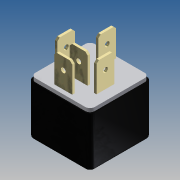
# Autodesk Inventor part: 24v relay
Saved by Autodesk Inventor 2015 SP1 (Build 190203100, 203)
## iProperties
Created: 2015-01-28
Part Number: 24v relay
Material: Acetal Resin, Black
Document SubType Name: Modeling
Designer: kevin.shaw
Mass: 21.4248 g
Surface Area: 35.5827 cm^2
Volume: 15.035 cm^3
Density: 1.425 g/cm^3
Appearance: Smooth - Black
Author: kevin.shaw
Autodesk Inventor part; units mm, degrees
note: some values were not read from the file. Chosen so that the rebuilt part matches the saved one: direction of "Emboss1".
(part 1 of 2)
ref_plane "YZ Plane" through (0, 0, 0) normal (1, 0, 0) x (0, 1, 0)
ref_plane "XZ Plane" through (0, 0, 0) normal (0, 1, 0) x (-1, 0, 0)
ref_plane "XY Plane" through (0, 0, 0) normal (0, 0, 1) x (1, 0, 0)
sketch "Sketch1" plane through (0, 0, 0) normal (0, 0, 1) x (1, 0, 0)
  line L0 (13, -13) -> (-13, -13)
  line L1 (-13, -13) -> (-13, 13)
  line L2 (-13, 13) -> (13, 13)
  line L3 (13, 13) -> (13, -13)
  line L4 (13, -13) -> (-13, 13) construction
  line L5 (-13, -13) -> (13, 13) construction
  point P0 (0, 0)
  dimension "d0" = 26
  dimension "d1" = 26
  constraints: 12 end point, 2 midpoint, 2 parallel, 1 horizontal, 1 perpendicular
  measures "d0" distance of L1.end L2.end
  measures "d1" distance of L0.end L1.end
extrude "Extrusion1" add sketch "Sketch1" along normal blind 21
sketch "Sketch2" plane through (0, 0, 21) normal (0, 0, 1) x (1, 0, 0)
  line L0 (-13, -13) -> (13, -13) projected
  line L1 (13, -13) -> (13, 13) projected
  line L2 (13, 13) -> (-13, 13) projected
  line L3 (-13, 13) -> (-13, -13) projected
  line L4 (-12.5, 12.5) -> (12.5, 12.5)
  line L5 (12.5, 12.5) -> (12.5, -12.5)
  line L6 (12.5, -12.5) -> (-12.5, -12.5)
  line L7 (-12.5, -12.5) -> (-12.5, 12.5)
  point P0 (0, 0)
  dimension "d4" = 0.5
  constraints: 8 end point, 3 other
  measures "d4" distance between parallel lines of L4 L2
extrude "Extrusion2" add sketch "Sketch2" along normal blind 1.5 contours L4 L5 L6 L7
fillet "Fillet1" radius 2 8 edges at (-13, -13, 10.5) (-13, 13, 10.5) (13, 13, 10.5) (13, -13, 10.5) (12.5, -12.5, 21.75) (-12.5, -12.5, 21.75) (-12.5, 12.5, 21.75) (12.5, 12.5, 21.75)
fillet "Fillet2" radius 1 8 edges at (12.4142, -12.4142, 0) (0, -13, 0) (-12.4142, -12.4142, 0) (-13, 0, 0) (-12.4142, 12.4142, 0) (0, 13, 0) (12.4142, 12.4142, 0) (13, 0, 0)
sketch "Sketch3" plane through (-11, 13, 21) normal (0, 1, 0) x (1, 0, 0)
  line L0 (1.1479, 5.5323) -> (24.0992, 5.5323) construction
  line L1 (24.0992, 5.5323) -> (24.0992, 1.9586) construction
  line L2 (24.0992, 1.9586) -> (1.1479, 1.9586) construction
  line L3 (1.1479, 1.9586) -> (1.1479, 5.5323) construction
  line L4 (3.2512, 2.4181) -> (1.3703, 2.4181)
  line L5 (1.3703, 2.4181) -> (1.3703, 2.8506)
  spline S0 degree 2 poles (1.3703, 2.8506) (1.573, 3.0409) (1.9338, 3.3944) (2.1069, 3.5847) knots 0 0 0 1 2 2 2
  spline S1 degree 2 poles (2.1069, 3.5847) (2.4554, 3.9678) (2.7099, 4.4275) (2.7099, 4.6722) knots 0 0 0 1 2 2 2
  spline S2 degree 2 poles (2.7099, 4.6722) (2.7099, 4.8007) (2.6308, 4.9935) (2.5592, 5.0553) knots 0 0 0 1 2 2 2
  spline S3 degree 2 poles (2.5592, 5.0553) (2.4875, 5.1171) (2.2996, 5.1789) (2.186, 5.1789) knots 0 0 0 1 2 2 2
  spline S4 degree 2 poles (2.186, 5.1789) (2.0772, 5.1789) (1.8548, 5.1245) (1.7534, 5.0825) knots 0 0 0 1 2 2 2
  spline S5 degree 2 poles (1.7534, 5.0825) (1.6669, 5.0479) (1.5063, 4.949) (1.4568, 4.9144) knots 0 0 0 1 2 2 2
  line L6 (1.4568, 4.9144) -> (1.4346, 4.9144)
  line L7 (1.4346, 4.9144) -> (1.4346, 5.3494)
  spline S6 degree 2 poles (1.4346, 5.3494) (1.5606, 5.4112) (2.0129, 5.5323) (2.2156, 5.5323) knots 0 0 0 1 2 2 2
  spline S7 degree 2 poles (2.2156, 5.5323) (2.6432, 5.5323) (3.1252, 5.08) (3.1252, 4.6945) knots 0 0 0 1 2 2 2
  spline S8 degree 2 poles (3.1252, 4.6945) (3.1252, 4.514) (3.0411, 4.2125) (2.967, 4.084) knots 0 0 0 1 2 2 2
  spline S9 degree 2 poles (2.967, 4.084) (2.8928, 3.9505) (2.6778, 3.6885) (2.5592, 3.5625) knots 0 0 0 1 2 2 2
  spline S10 degree 2 poles (2.5592, 3.5625) (2.3664, 3.3524) (1.8943, 2.9025) (1.7534, 2.7715) knots 0 0 0 1 2 2 2
  line L8 (1.7534, 2.7715) -> (3.2512, 2.7715)
  line L9 (3.2512, 2.7715) -> (3.2512, 2.4181)
  line L10 (5.6215, 3.4661) -> (5.2582, 3.4661)
  line L11 (5.2582, 3.4661) -> (5.2582, 2.4181)
  line L12 (5.2582, 2.4181) -> (4.8652, 2.4181)
  line L13 (4.8652, 2.4181) -> (4.8652, 3.4661)
  line L14 (4.8652, 3.4661) -> (3.5182, 3.4661)
  line L15 (3.5182, 3.4661) -> (3.5182, 3.8961)
  line L16 (3.5182, 3.8961) -> (4.8825, 5.4681)
  line L17 (4.8825, 5.4681) -> (5.2582, 5.4681)
  line L18 (5.2582, 5.4681) -> (5.2582, 3.7948)
  line L19 (5.2582, 3.7948) -> (5.6215, 3.7948)
  line L20 (5.6215, 3.7948) -> (5.6215, 3.4661)
  line L21 (4.8652, 3.7948) -> (4.8652, 4.9861)
  line L22 (4.8652, 4.9861) -> (3.8395, 3.7948)
  line L23 (3.8395, 3.7948) -> (4.8652, 3.7948)
  line L24 (7.8015, 4.7068) -> (6.9389, 2.4181)
  line L25 (6.9389, 2.4181) -> (6.5929, 2.4181)
  line L26 (6.5929, 2.4181) -> (5.7377, 4.7068)
  line L27 (5.7377, 4.7068) -> (6.1554, 4.7068)
  line L28 (6.1554, 4.7068) -> (6.7807, 2.9445)
  line L29 (6.7807, 2.9445) -> (7.4011, 4.7068)
  line L30 (7.4011, 4.7068) -> (7.8015, 4.7068)
  line L31 (11.7932, 2.4181) -> (11.2667, 2.4181)
  line L32 (11.2667, 2.4181) -> (10.3028, 3.6317)
  line L33 (10.3028, 3.6317) -> (9.8381, 3.6317)
  line L34 (9.8381, 3.6317) -> (9.8381, 2.4181)
  line L35 (9.8381, 2.4181) -> (9.4328, 2.4181)
  line L36 (9.4328, 2.4181) -> (9.4328, 5.4681)
  line L37 (9.4328, 5.4681) -> (10.2188, 5.4681)
  spline S11 degree 2 poles (10.2188, 5.4681) (10.4808, 5.4681) (10.8342, 5.4112) (10.9949, 5.3074) knots 0 0 0 1 2 2 2
  spline S12 degree 2 poles (10.9949, 5.3074) (11.1555, 5.2036) (11.3409, 4.8798) (11.3409, 4.6401) knots 0 0 0 1 2 2 2
  spline S13 degree 2 poles (11.3409, 4.6401) (11.3409, 4.3064) (10.9998, 3.8541) (10.7082, 3.7454) knots 0 0 0 1 2 2 2
  line L38 (10.7082, 3.7454) -> (11.7932, 2.4181)
  spline S14 degree 2 poles (10.9182, 4.608) (10.9182, 4.7414) (10.8243, 4.9466) (10.7255, 5.0133) knots 0 0 0 1 2 2 2
  spline S15 degree 2 poles (10.7255, 5.0133) (10.639, 5.0702) (10.4091, 5.1171) (10.241, 5.1171) knots 0 0 0 1 2 2 2
  line L39 (10.241, 5.1171) -> (9.8381, 5.1171)
  line L40 (9.8381, 5.1171) -> (9.8381, 3.9703)
  line L41 (9.8381, 3.9703) -> (10.1941, 3.9703)
  spline S16 degree 2 poles (10.1941, 3.9703) (10.3695, 3.9703) (10.6488, 4.0321) (10.7452, 4.1285) knots 0 0 0 1 2 2 2
  spline S17 degree 2 poles (10.7452, 4.1285) (10.8342, 4.2125) (10.9182, 4.4498) (10.9182, 4.608) knots 0 0 0 1 2 2 2
  line L42 (12.0354, 2.4181) -> (12.0354, 5.4681)
  line L43 (12.0354, 5.4681) -> (13.9435, 5.4681)
  line L44 (13.9435, 5.4681) -> (13.9435, 5.1072)
  line L45 (13.9435, 5.1072) -> (12.4408, 5.1072)
  line L46 (12.4408, 5.1072) -> (12.4408, 4.2718)
  line L47 (12.4408, 4.2718) -> (13.8422, 4.2718)
  line L48 (13.8422, 4.2718) -> (13.8422, 3.911)
  line L49 (13.8422, 3.911) -> (12.4408, 3.911)
  line L50 (12.4408, 3.911) -> (12.4408, 2.7789)
  line L51 (12.4408, 2.7789) -> (13.9435, 2.7789)
  line L52 (13.9435, 2.7789) -> (13.9435, 2.4181)
  line L53 (13.9435, 2.4181) -> (12.0354, 2.4181)
  line L54 (16.1556, 2.4181) -> (14.3884, 2.4181)
  line L55 (14.3884, 2.4181) -> (14.3884, 5.4681)
  line L56 (14.3884, 5.4681) -> (14.7938, 5.4681)
  line L57 (14.7938, 5.4681) -> (14.7938, 2.7789)
  line L58 (14.7938, 2.7789) -> (16.1556, 2.7789)
  line L59 (16.1556, 2.7789) -> (16.1556, 2.4181)
  line L60 (16.1458, 2.4181) -> (17.174, 5.4681)
  line L61 (17.174, 5.4681) -> (17.6732, 5.4681)
  line L62 (17.6732, 5.4681) -> (18.7014, 2.4181)
  line L63 (18.7014, 2.4181) -> (18.2738, 2.4181)
  line L64 (18.2738, 2.4181) -> (17.997, 3.2708)
  line L65 (17.997, 3.2708) -> (16.8329, 3.2708)
  line L66 (16.8329, 3.2708) -> (16.5561, 2.4181)
  line L67 (16.5561, 2.4181) -> (16.1458, 2.4181)
  line L68 (17.8858, 3.6168) -> (17.4137, 5.0528)
  line L69 (17.4137, 5.0528) -> (16.9441, 3.6168)
  line L70 (16.9441, 3.6168) -> (17.8858, 3.6168)
  line L71 (21.1261, 5.4681) -> (20.0954, 3.7676)
  line L72 (20.0954, 3.7676) -> (20.0954, 2.4181)
  line L73 (20.0954, 2.4181) -> (19.6901, 2.4181)
  line L74 (19.6901, 2.4181) -> (19.6901, 3.7256)
  line L75 (19.6901, 3.7256) -> (18.6594, 5.4681)
  line L76 (18.6594, 5.4681) -> (19.1093, 5.4681)
  line L77 (19.1093, 5.4681) -> (19.8952, 4.126)
  line L78 (19.8952, 4.126) -> (20.696, 5.4681)
  line L79 (20.696, 5.4681) -> (21.1261, 5.4681)
  point P0 (11, 21)
  constraints: 2 other
emboss "Emboss1" sketch "Sketch3" operation cut depth 0.1 direction (0, -1, 0)
sketch "Sketch4" plane through (0, 0, 22.5) normal (0, 0, 1) x (1, 0, 0)
  line L0 (-1.75, 11.75) -> (-0.75, 11.75)
  line L1 (-0.75, 11.75) -> (-0.75, 4.25)
  line L2 (-0.75, 4.25) -> (-1.75, 4.25)
  line L3 (-1.75, 4.25) -> (-1.75, 11.75)
  line L4 (-4.25, -3.25) -> (3.25, -3.25)
  line L5 (3.25, -3.25) -> (3.25, -4.25)
  line L6 (3.25, -4.25) -> (-4.25, -4.25)
  line L7 (-4.25, -4.25) -> (-4.25, -3.25)
  line L8 (-4.25, -9.75) -> (3.25, -9.75)
  line L9 (3.25, -9.75) -> (3.25, -10.75)
  line L10 (3.25, -10.75) -> (-4.25, -10.75)
  line L11 (-4.25, -10.75) -> (-4.25, -9.75)
  line L12 (-11, 13) -> (11, 13) projected
  line L13 (13, -11) -> (13, 11) projected
  line L14 (-9.25, 2) -> (-8.25, 2)
  line L15 (-8.25, 2) -> (-8.25, -5.5)
  line L16 (-8.25, -5.5) -> (-9.25, -5.5)
  line L17 (-9.25, -5.5) -> (-9.25, 2)
  line L18 (7.25, 2) -> (8.25, 2)
  line L19 (8.25, 2) -> (8.25, -5.5)
  line L20 (8.25, -5.5) -> (7.25, -5.5)
  line L21 (7.25, -5.5) -> (7.25, 2)
  line L22 (-13, 11) -> (-13, -11) projected
  point P0 (0, 0)
  dimension "d11" = 7.5
  dimension "d12" = 1
  dimension "d13" = 5.5
  dimension "d14" = 7.5
  dimension "d15" = 23.75
  dimension "d19" = 2.5
  dimension "d70" = 15.5
  dimension "d71" = 11.25
  dimension "d72" = 4
  dimension "d73" = 11
  constraints: 40 end point, 10 parallel, 8 equal length, 5 horizontal, 5 perpendicular, 2 point on line
  measures "d11" distance of L5.end L6.end
  measures "d12" distance of L6.end L4.start
  measures "d13" distance between parallel lines of L6 L8
  measures "d14" distance between parallel lines of L2 L4
  measures "d15" distance between parallel lines of L12 L10
  measures "d19" distance between parallel lines of L3 L7
  measures "d70" distance between parallel lines of L21 L15
  measures "d71" distance between parallel lines of L3 L22
  measures "d72" distance between parallel lines of L15 L7
  measures "d73" distance between parallel lines of L12 L18
extrude "Extrusion3" add sketch "Sketch4" along normal blind 12
chamfer "Chamfer1" distance 1 angle 45 10 edges at (-4.25, -10.25, 34.5) (3.25, -10.25, 34.5) (-4.25, -3.75, 34.5) (3.25, -3.75, 34.5) (-1.25, 4.25, 34.5) (-1.25, 11.75, 34.5) (-8.75, -5.5, 34.5) (-8.75, 2, 34.5) (7.75, -5.5, 34.5) (7.75, 2, 34.5)
hole "Hole1" at (-0.5, -10.75, 29.5) direction (0, 1, 0) diameter 2 depth 2 tip angle 118
hole "Hole2" at (-0.5, -4.25, 29.5) direction (0, 1, 0) diameter 2 depth 2 tip angle 118
hole "Hole5" at (-0.75, 8, 29.5) direction (-1, 0, 0) diameter 2 depth 2 tip angle 118
hole "Hole6" at (8.25, -1.75, 29.5) direction (-1, 0, 0) diameter 2 depth 2 tip angle 118
hole "Hole7" at (-8.25, -1.75, 29.5) direction (-1, 0, 0) diameter 2 depth 2 tip angle 118
sketch "Sketch5" plane through (0, 0, 0) normal (0, 0, -1) x (-1, 0, 0)
  line L0 (5, -5) -> (-2, -5)
  line L1 (-2, -5) -> (-2, -1)
  line L2 (-2, -1) -> (5, -1)
  line L3 (5, -1) -> (5, -5)
  line L4 (-13, 11) -> (-13, -11) projected
  line L5 (11, 13) -> (-11, 13) projected
  line L6 (3, -5) -> (0, -1)
  line L7 (8, -3) -> (6, -3)
  line L8 (7, -2.9) -> (7, 0.5)
  line L9 (7, 0.5) -> (0, 0.5)
  line L10 (7, -3) -> (6, -4.7321)
  line L11 (8, -4.7321) -> (7, -3)
  line L12 (3, -6.5) -> (7, -6.5)
  line L13 (7, -6.5) -> (7, -4.7321)
  line L14 (-2, -3) -> (-4, -3)
  line L15 (-4.9676, -7.9116) -> (-3.9257, -2.0028)
  line L16 (-3.9257, -2.0028) -> (-3.9257, 2.9972)
  line L17 (-4.8794, -7.4116) -> (-5.8794, -7.4116)
  line L18 (-5.8794, -7.4116) -> (-5.8794, -9.4116)
  line L19 (-3.3794, -7.4116) -> (-2.3794, -7.4116)
  line L20 (-2.3794, -7.4116) -> (-2.3794, -9.4116)
  line L21 (4.1535, -10.1598) -> (1.8061, -10.1598) construction
  line L22 (1.8061, -10.1598) -> (1.8061, -8.2773) construction
  line L23 (1.8061, -8.2773) -> (4.1535, -8.2773) construction
  line L24 (4.1535, -8.2773) -> (4.1535, -10.1598) construction
  line L25 (-1.2772, -11.3985) -> (-3.5284, -11.3985) construction
  line L26 (-3.5284, -11.3985) -> (-3.5284, -9.8304) construction
  line L27 (-3.5284, -9.8304) -> (-1.2772, -9.8304) construction
  line L28 (-1.2772, -9.8304) -> (-1.2772, -11.3985) construction
  line L29 (1.1157, 2.3398) -> (-1.1355, 2.3398) construction
  line L30 (-1.1355, 2.3398) -> (-1.1355, 3.9079) construction
  line L31 (-1.1355, 3.9079) -> (1.1157, 3.9079) construction
  line L32 (1.1157, 3.9079) -> (1.1157, 2.3398) construction
  line L33 (-2.7765, 3.4766) -> (-5.0277, 3.4766) construction
  line L34 (-5.0277, 3.4766) -> (-5.0277, 5.0398) construction
  line L35 (-5.0277, 5.0398) -> (-2.7765, 5.0398) construction
  line L36 (-2.7765, 5.0398) -> (-2.7765, 3.4766) construction
  line L37 (-4.4694, -11.3822) -> (-7.8036, -11.3822) construction
  line L38 (-7.8036, -11.3822) -> (-7.8036, -9.8141) construction
  line L39 (-7.8036, -9.8141) -> (-4.4694, -9.8141) construction
  line L40 (-4.4694, -9.8141) -> (-4.4694, -11.3822) construction
  line L41 (7.1, -4.7321) -> (7.1, -6.6)
  line L42 (7.1, -6.6) -> (3, -6.6)
  line L43 (8, -3) -> (8, -2.9)
  line L44 (6, -3) -> (6, -2.9)
  line L45 (7.1, -2.9) -> (7.1, 0.6)
  line L46 (7.1, 0.6) -> (0, 0.6)
  line L47 (8, -2.9) -> (7.1, -2.9)
  line L48 (7, -2.9) -> (6, -2.9)
  line L49 (-0.125, -1) -> (2.875, -5)
  line L50 (0, 2) -> (-0.1, 2)
  line L51 (3, -8) -> (2.9, -8)
  line L52 (5.1, -0.9) -> (-2.1, -0.9)
  line L53 (-2.1, -0.9) -> (-2.1, -5.1)
  line L54 (-2.1, -5.1) -> (5.1, -5.1)
  line L55 (5.1, -5.1) -> (5.1, -0.9)
  line L56 (-2.4794, -9.4116) -> (-2.4794, -7.5116)
  line L57 (-2.4794, -7.5116) -> (-3.3794, -7.5116)
  line L58 (-2.3794, -9.4116) -> (-2.4794, -9.4116)
  line L59 (-3.3794, -7.5116) -> (-3.3794, -7.4116)
  line L60 (-5.9794, -9.4116) -> (-5.9794, -7.3116)
  line L61 (-5.9794, -7.3116) -> (-4.8618, -7.3116)
  line L62 (-5.8794, -9.4116) -> (-5.9794, -9.4116)
  line L63 (-4.8691, -7.929) -> (-3.8257, -2.0115)
  line L64 (-3.8257, -2.0115) -> (-3.8257, 2.9972)
  line L65 (-4.8691, -7.929) -> (-4.9676, -7.9116)
  line L66 (-3.8257, 2.9972) -> (-3.9257, 2.9972)
  line L67 (0, 0.6) -> (0, 2)
  line L68 (3, -6.6) -> (3, -8)
  line L69 (6, -4.7321) -> (7, -4.7321)
  line L70 (7.1, -4.7321) -> (8, -4.7321)
  line L71 (3, -5.2) -> (2.9, -5.2)
  line L72 (2.9, -5.2) -> (2.9, -8)
  line L73 (3, -5.2) -> (3, -6.5)
  line L74 (0, -0.8) -> (-0.1, -0.8)
  line L75 (-0.1, 2) -> (-0.1, -0.8)
  line L76 (0, -1) -> (0, -0.9)
  line L77 (0, -0.8) -> (0, 0.5)
  line L78 (-2, -3.1) -> (-4.0176, -3.1)
  spline S0 degree 2 poles (-5.0322, -9.8141) (-4.9203, -9.8141) (-4.7368, -9.881) (-4.6724, -9.943) knots 0 0 0 1 2 2 2
  spline S1 degree 2 poles (-4.6724, -9.943) (-4.6091, -10.0038) (-4.5435, -10.1691) (-4.5435, -10.2627) knots 0 0 0 1 2 2 2
  spline S2 degree 2 poles (-4.5435, -10.2627) (-4.5435, -10.3842) (-4.6736, -10.5884) (-4.7976, -10.6492) knots 0 0 0 1 2 2 2
  line L79 (-4.7976, -10.6492) -> (-4.7976, -10.6553)
  spline S3 degree 2 poles (-4.7976, -10.6553) (-4.6869, -10.7197) (-4.58, -10.8729) (-4.58, -10.9872) knots 0 0 0 1 2 2 2
  spline S4 degree 2 poles (-4.58, -10.9872) (-4.58, -11.1561) (-4.8352, -11.3822) (-5.0322, -11.3822) knots 0 0 0 1 2 2 2
  spline S5 degree 2 poles (-5.0322, -11.3822) (-5.2364, -11.3822) (-5.4831, -11.1683) (-5.4831, -11.0005) knots 0 0 0 1 2 2 2
  spline S6 degree 2 poles (-5.4831, -11.0005) (-5.4831, -10.8996) (-5.3652, -10.7027) (-5.2546, -10.6468) knots 0 0 0 1 2 2 2
  line L80 (-5.2546, -10.6468) -> (-5.2546, -10.6407)
  spline S7 degree 2 poles (-5.2546, -10.6407) (-5.3859, -10.5799) (-5.5208, -10.4049) (-5.5208, -10.2663) knots 0 0 0 1 2 2 2
  spline S8 degree 2 poles (-5.5208, -10.2663) (-5.5208, -10.0743) (-5.2412, -9.8141) (-5.0322, -9.8141) knots 0 0 0 1 2 2 2
  spline S9 degree 2 poles (-5.3142, -10.2469) (-5.3142, -10.3393) (-5.2412, -10.4487) (-5.1379, -10.5046) knots 0 0 0 1 2 2 2
  spline S10 degree 2 poles (-5.1379, -10.5046) (-5.1039, -10.524) (-4.9896, -10.569) (-4.9179, -10.5982) knots 0 0 0 1 2 2 2
  spline S11 degree 2 poles (-4.9179, -10.5982) (-4.8352, -10.5435) (-4.7465, -10.3806) (-4.7465, -10.2773) knots 0 0 0 1 2 2 2
  spline S12 degree 2 poles (-4.7465, -10.2773) (-4.7465, -10.1411) (-4.9106, -9.9637) (-5.0346, -9.9637) knots 0 0 0 1 2 2 2
  spline S13 degree 2 poles (-5.0346, -9.9637) (-5.161, -9.9637) (-5.3142, -10.1156) (-5.3142, -10.2469) knots 0 0 0 1 2 2 2
  spline S14 degree 2 poles (-5.2862, -10.9981) (-5.2862, -11.099) (-5.1513, -11.2339) (-5.0309, -11.2339) knots 0 0 0 1 2 2 2
  spline S15 degree 2 poles (-5.0309, -11.2339) (-4.9215, -11.2339) (-4.7818, -11.1136) (-4.7818, -11.0102) knots 0 0 0 1 2 2 2
  spline S16 degree 2 poles (-4.7818, -11.0102) (-4.7818, -10.9361) (-4.8535, -10.8328) (-4.9252, -10.7914) knots 0 0 0 1 2 2 2
  spline S17 degree 2 poles (-4.9252, -10.7914) (-4.9556, -10.7744) (-5.0844, -10.7149) (-5.1367, -10.6978) knots 0 0 0 1 2 2 2
  spline S18 degree 2 poles (-5.1367, -10.6978) (-5.2242, -10.7647) (-5.2862, -10.9069) (-5.2862, -10.9981) knots 0 0 0 1 2 2 2
  line L81 (-6.6464, -11.1233) -> (-5.9973, -9.8482)
  line L82 (-5.9973, -9.8482) -> (-5.7834, -9.8482)
  line L83 (-5.7834, -9.8482) -> (-6.4689, -11.1719)
  line L84 (-6.4689, -11.1719) -> (-5.6946, -11.1719)
  line L85 (-5.6946, -11.1719) -> (-5.6946, -11.3482)
  line L86 (-5.6946, -11.3482) -> (-6.6464, -11.3482)
  line L87 (-6.6464, -11.3482) -> (-6.6464, -11.1233)
  spline S19 degree 2 poles (-7.4852, -9.9673) (-7.4621, -9.9503) (-7.3843, -9.8895) (-7.3478, -9.8713) knots 0 0 0 1 2 2 2
  spline S20 degree 2 poles (-7.3478, -9.8713) (-7.298, -9.8445) (-7.2044, -9.8166) (-7.1193, -9.8166) knots 0 0 0 1 2 2 2
  spline S21 degree 2 poles (-7.1193, -9.8166) (-7.05, -9.8166) (-6.9248, -9.8688) (-6.8774, -9.9162) knots 0 0 0 1 2 2 2
  spline S22 degree 2 poles (-6.8774, -9.9162) (-6.8324, -9.9624) (-6.7777, -10.0986) (-6.7777, -10.1739) knots 0 0 0 1 2 2 2
  spline S23 degree 2 poles (-6.7777, -10.1739) (-6.7777, -10.2906) (-6.8762, -10.456) (-6.9831, -10.5034) knots 0 0 0 1 2 2 2
  spline S24 degree 2 poles (-6.9831, -10.5034) (-7.0779, -10.5471) (-7.3356, -10.5799) (-7.4852, -10.5884) knots 0 0 0 1 2 2 2
  line L88 (-7.4852, -10.5884) -> (-7.4852, -10.6249)
  spline S25 degree 2 poles (-7.4852, -10.6249) (-7.4852, -10.6906) (-7.445, -10.772) (-7.4086, -10.7951) knots 0 0 0 1 2 2 2
  spline S26 degree 2 poles (-7.4086, -10.7951) (-7.3721, -10.8182) (-7.2676, -10.8328) (-7.2117, -10.8328) knots 0 0 0 1 2 2 2
  spline S27 degree 2 poles (-7.2117, -10.8328) (-7.146, -10.8328) (-6.9685, -10.7939) (-6.8798, -10.7562) knots 0 0 0 1 2 2 2
  line L89 (-6.8798, -10.7562) -> (-6.8689, -10.7562)
  line L90 (-6.8689, -10.7562) -> (-6.8689, -10.9495)
  spline S28 degree 2 poles (-6.8689, -10.9495) (-6.9211, -10.9641) (-7.1168, -11.0005) (-7.2129, -11.0005) knots 0 0 0 1 2 2 2
  spline S29 degree 2 poles (-7.2129, -11.0005) (-7.3296, -11.0005) (-7.4888, -10.9641) (-7.552, -10.9166) knots 0 0 0 1 2 2 2
  spline S30 degree 2 poles (-7.552, -10.9166) (-7.614, -10.8705) (-7.6748, -10.7234) (-7.6748, -10.6176) knots 0 0 0 1 2 2 2
  line L91 (-7.6748, -10.6176) -> (-7.6748, -9.8482)
  line L92 (-7.6748, -9.8482) -> (-7.4852, -9.8482)
  line L93 (-7.4852, -9.8482) -> (-7.4852, -9.9673)
  line L94 (-7.4852, -10.1253) -> (-7.4852, -10.4377)
  spline S31 degree 2 poles (-7.4852, -10.4377) (-7.4171, -10.4316) (-7.2117, -10.411) (-7.1472, -10.3915) knots 0 0 0 1 2 2 2
  spline S32 degree 2 poles (-7.1472, -10.3915) (-7.0719, -10.3684) (-6.9734, -10.2724) (-6.9734, -10.1873) knots 0 0 0 1 2 2 2
  spline S33 degree 2 poles (-6.9734, -10.1873) (-6.9734, -10.0901) (-7.0828, -9.9916) (-7.1873, -9.9916) knots 0 0 0 1 2 2 2
  spline S34 degree 2 poles (-7.1873, -9.9916) (-7.2761, -9.9916) (-7.4219, -10.0682) (-7.4852, -10.1253) knots 0 0 0 1 2 2 2
  spline S35 degree 2 poles (-1.84, -9.8304) (-1.7282, -9.8304) (-1.5446, -9.8973) (-1.4802, -9.9593) knots 0 0 0 1 2 2 2
  spline S36 degree 2 poles (-1.4802, -9.9593) (-1.417, -10.02) (-1.3513, -10.1854) (-1.3513, -10.279) knots 0 0 0 1 2 2 2
  spline S37 degree 2 poles (-1.3513, -10.279) (-1.3513, -10.4005) (-1.4814, -10.6047) (-1.6054, -10.6655) knots 0 0 0 1 2 2 2
  line L95 (-1.6054, -10.6655) -> (-1.6054, -10.6716)
  spline S38 degree 2 poles (-1.6054, -10.6716) (-1.4948, -10.736) (-1.3878, -10.8892) (-1.3878, -11.0034) knots 0 0 0 1 2 2 2
  spline S39 degree 2 poles (-1.3878, -11.0034) (-1.3878, -11.1724) (-1.6431, -11.3985) (-1.84, -11.3985) knots 0 0 0 1 2 2 2
  spline S40 degree 2 poles (-1.84, -11.3985) (-2.0442, -11.3985) (-2.291, -11.1845) (-2.291, -11.0168) knots 0 0 0 1 2 2 2
  spline S41 degree 2 poles (-2.291, -11.0168) (-2.291, -10.9159) (-2.1731, -10.719) (-2.0624, -10.6631) knots 0 0 0 1 2 2 2
  line L96 (-2.0624, -10.6631) -> (-2.0624, -10.657)
  spline S42 degree 2 poles (-2.0624, -10.657) (-2.1937, -10.5962) (-2.3286, -10.4212) (-2.3286, -10.2826) knots 0 0 0 1 2 2 2
  spline S43 degree 2 poles (-2.3286, -10.2826) (-2.3286, -10.0905) (-2.0491, -9.8304) (-1.84, -9.8304) knots 0 0 0 1 2 2 2
  spline S44 degree 2 poles (-2.122, -10.2631) (-2.122, -10.3555) (-2.0491, -10.4649) (-1.9457, -10.5208) knots 0 0 0 1 2 2 2
  spline S45 degree 2 poles (-1.9457, -10.5208) (-1.9117, -10.5403) (-1.7974, -10.5853) (-1.7257, -10.6144) knots 0 0 0 1 2 2 2
  spline S46 degree 2 poles (-1.7257, -10.6144) (-1.6431, -10.5597) (-1.5543, -10.3969) (-1.5543, -10.2935) knots 0 0 0 1 2 2 2
  spline S47 degree 2 poles (-1.5543, -10.2935) (-1.5543, -10.1574) (-1.7184, -9.9799) (-1.8424, -9.9799) knots 0 0 0 1 2 2 2
  spline S48 degree 2 poles (-1.8424, -9.9799) (-1.9688, -9.9799) (-2.122, -10.1319) (-2.122, -10.2631) knots 0 0 0 1 2 2 2
  spline S49 degree 2 poles (-2.094, -11.0144) (-2.094, -11.1153) (-1.9591, -11.2502) (-1.8388, -11.2502) knots 0 0 0 1 2 2 2
  spline S50 degree 2 poles (-1.8388, -11.2502) (-1.7294, -11.2502) (-1.5896, -11.1298) (-1.5896, -11.0265) knots 0 0 0 1 2 2 2
  spline S51 degree 2 poles (-1.5896, -11.0265) (-1.5896, -10.9524) (-1.6613, -10.849) (-1.733, -10.8077) knots 0 0 0 1 2 2 2
  spline S52 degree 2 poles (-1.733, -10.8077) (-1.7634, -10.7907) (-1.8923, -10.7311) (-1.9445, -10.7141) knots 0 0 0 1 2 2 2
  spline S53 degree 2 poles (-1.9445, -10.7141) (-2.032, -10.781) (-2.094, -10.9232) (-2.094, -11.0144) knots 0 0 0 1 2 2 2
  line L97 (-3.4543, -11.1396) -> (-2.8051, -9.8644)
  line L98 (-2.8051, -9.8644) -> (-2.5912, -9.8644)
  line L99 (-2.5912, -9.8644) -> (-3.2768, -11.1882)
  line L100 (-3.2768, -11.1882) -> (-2.5025, -11.1882)
  line L101 (-2.5025, -11.1882) -> (-2.5025, -11.3644)
  line L102 (-2.5025, -11.3644) -> (-3.4543, -11.3644)
  line L103 (-3.4543, -11.3644) -> (-3.4543, -11.1396)
  spline S54 degree 2 poles (3.5907, -8.5918) (3.7025, -8.5918) (3.8861, -8.6586) (3.9505, -8.7206) knots 0 0 0 1 2 2 2
  spline S55 degree 2 poles (3.9505, -8.7206) (4.0137, -8.7814) (4.0793, -8.9467) (4.0793, -9.0403) knots 0 0 0 1 2 2 2
  spline S56 degree 2 poles (4.0793, -9.0403) (4.0793, -9.1619) (3.9493, -9.3661) (3.8253, -9.4269) knots 0 0 0 1 2 2 2
  line L104 (3.8253, -9.4269) -> (3.8253, -9.4329)
  spline S57 degree 2 poles (3.8253, -9.4329) (3.9359, -9.4974) (4.0429, -9.6505) (4.0429, -9.7648) knots 0 0 0 1 2 2 2
  spline S58 degree 2 poles (4.0429, -9.7648) (4.0429, -9.9338) (3.7876, -10.1598) (3.5907, -10.1598) knots 0 0 0 1 2 2 2
  spline S59 degree 2 poles (3.5907, -10.1598) (3.3865, -10.1598) (3.1397, -9.9459) (3.1397, -9.7782) knots 0 0 0 1 2 2 2
  spline S60 degree 2 poles (3.1397, -9.7782) (3.1397, -9.6773) (3.2576, -9.4803) (3.3682, -9.4244) knots 0 0 0 1 2 2 2
  line L105 (3.3682, -9.4244) -> (3.3682, -9.4184)
  spline S61 degree 2 poles (3.3682, -9.4184) (3.2369, -9.3576) (3.102, -9.1825) (3.102, -9.044) knots 0 0 0 1 2 2 2
  spline S62 degree 2 poles (3.102, -9.044) (3.102, -8.8519) (3.3816, -8.5918) (3.5907, -8.5918) knots 0 0 0 1 2 2 2
  spline S63 degree 2 poles (3.3087, -9.0245) (3.3087, -9.1169) (3.3816, -9.2263) (3.4849, -9.2822) knots 0 0 0 1 2 2 2
  spline S64 degree 2 poles (3.4849, -9.2822) (3.519, -9.3017) (3.6332, -9.3466) (3.7049, -9.3758) knots 0 0 0 1 2 2 2
  spline S65 degree 2 poles (3.7049, -9.3758) (3.7876, -9.3211) (3.8763, -9.1582) (3.8763, -9.0549) knots 0 0 0 1 2 2 2
  spline S66 degree 2 poles (3.8763, -9.0549) (3.8763, -8.9188) (3.7122, -8.7413) (3.5882, -8.7413) knots 0 0 0 1 2 2 2
  spline S67 degree 2 poles (3.5882, -8.7413) (3.4618, -8.7413) (3.3087, -8.8932) (3.3087, -9.0245) knots 0 0 0 1 2 2 2
  spline S68 degree 2 poles (3.3366, -9.7757) (3.3366, -9.8766) (3.4715, -10.0115) (3.5919, -10.0115) knots 0 0 0 1 2 2 2
  spline S69 degree 2 poles (3.5919, -10.0115) (3.7013, -10.0115) (3.8411, -9.8912) (3.8411, -9.7879) knots 0 0 0 1 2 2 2
  spline S70 degree 2 poles (3.8411, -9.7879) (3.8411, -9.7137) (3.7694, -9.6104) (3.6976, -9.5691) knots 0 0 0 1 2 2 2
  spline S71 degree 2 poles (3.6976, -9.5691) (3.6672, -9.5521) (3.5384, -9.4925) (3.4861, -9.4755) knots 0 0 0 1 2 2 2
  spline S72 degree 2 poles (3.4861, -9.4755) (3.3986, -9.5423) (3.3366, -9.6846) (3.3366, -9.7757) knots 0 0 0 1 2 2 2
  spline S73 degree 2 poles (2.0092, -9.1023) (2.0092, -8.9941) (2.0785, -8.8094) (2.1417, -8.7413) knots 0 0 0 1 2 2 2
  spline S74 degree 2 poles (2.1417, -8.7413) (2.2049, -8.6732) (2.3933, -8.5942) (2.51, -8.5942) knots 0 0 0 1 2 2 2
  spline S75 degree 2 poles (2.51, -8.5942) (2.617, -8.5942) (2.8261, -8.6416) (2.9027, -8.6793) knots 0 0 0 1 2 2 2
  line L106 (2.9027, -8.6793) -> (2.9027, -8.892)
  line L107 (2.9027, -8.892) -> (2.8881, -8.892)
  spline S76 degree 2 poles (2.8881, -8.892) (2.865, -8.875) (2.7787, -8.8312) (2.7264, -8.8118) knots 0 0 0 1 2 2 2
  spline S77 degree 2 poles (2.7264, -8.8118) (2.6668, -8.7911) (2.5684, -8.768) (2.5064, -8.768) knots 0 0 0 1 2 2 2
  spline S78 degree 2 poles (2.5064, -8.768) (2.4456, -8.768) (2.3314, -8.8118) (2.29, -8.8592) knots 0 0 0 1 2 2 2
  spline S79 degree 2 poles (2.29, -8.8592) (2.2523, -8.9042) (2.2134, -9.0233) (2.2134, -9.1035) knots 0 0 0 1 2 2 2
  spline S80 degree 2 poles (2.2134, -9.1035) (2.2134, -9.1838) (2.2572, -9.2859) (2.2985, -9.3199) knots 0 0 0 1 2 2 2
  spline S81 degree 2 poles (2.2985, -9.3199) (2.3411, -9.3576) (2.4675, -9.3892) (2.5441, -9.3892) knots 0 0 0 1 2 2 2
  spline S82 degree 2 poles (2.5441, -9.3892) (2.6267, -9.3892) (2.7908, -9.3637) (2.8407, -9.3527) knots 0 0 0 1 2 2 2
  line L108 (2.8407, -9.3527) -> (2.8407, -10.1258)
  line L109 (2.8407, -10.1258) -> (2.0177, -10.1258)
  line L110 (2.0177, -10.1258) -> (2.0177, -9.9496)
  line L111 (2.0177, -9.9496) -> (2.6474, -9.9496)
  line L112 (2.6474, -9.9496) -> (2.6474, -9.5496)
  spline S83 degree 2 poles (2.6474, -9.5496) (2.6109, -9.5545) (2.5404, -9.5581) (2.5113, -9.5581) knots 0 0 0 1 2 2 2
  spline S84 degree 2 poles (2.5113, -9.5581) (2.3958, -9.5581) (2.2365, -9.5205) (2.1636, -9.4645) knots 0 0 0 1 2 2 2
  spline S85 degree 2 poles (2.1636, -9.4645) (2.0895, -9.4086) (2.0092, -9.2385) (2.0092, -9.1023) knots 0 0 0 1 2 2 2
  spline S86 degree 2 poles (-3.2907, 3.6505) (-3.236, 3.6505) (-3.1278, 3.6772) (-3.0755, 3.6979) knots 0 0 0 1 2 2 2
  spline S87 degree 2 poles (-3.0755, 3.6979) (-3.0269, 3.7185) (-2.9552, 3.7623) (-2.9272, 3.7817) knots 0 0 0 1 2 2 2
  line L113 (-2.9272, 3.7817) -> (-2.9151, 3.7817)
  line L114 (-2.9151, 3.7817) -> (-2.9151, 3.569)
  spline S88 degree 2 poles (-2.9151, 3.569) (-2.9807, 3.5338) (-3.2056, 3.4766) (-3.3065, 3.4766) knots 0 0 0 1 2 2 2
  spline S89 degree 2 poles (-3.3065, 3.4766) (-3.4086, 3.4766) (-3.5605, 3.518) (-3.6225, 3.5617) knots 0 0 0 1 2 2 2
  spline S90 degree 2 poles (-3.6225, 3.5617) (-3.6882, 3.6091) (-3.7563, 3.7465) (-3.7563, 3.8389) knots 0 0 0 1 2 2 2
  spline S91 degree 2 poles (-3.7563, 3.8389) (-3.7563, 3.9629) (-3.5934, 4.1501) (-3.4791, 4.1744) knots 0 0 0 1 2 2 2
  line L115 (-3.4791, 4.1744) -> (-3.4791, 4.1889)
  spline S92 degree 2 poles (-3.4791, 4.1889) (-3.5265, 4.1987) (-3.6347, 4.2424) (-3.6809, 4.2862) knots 0 0 0 1 2 2 2
  spline S93 degree 2 poles (-3.6809, 4.2862) (-3.7271, 4.3287) (-3.7854, 4.4649) (-3.7854, 4.5633) knots 0 0 0 1 2 2 2
  spline S94 degree 2 poles (-3.7854, 4.5633) (-3.7854, 4.6642) (-3.7161, 4.8356) (-3.6529, 4.9013) knots 0 0 0 1 2 2 2
  spline S95 degree 2 poles (-3.6529, 4.9013) (-3.5873, 4.9693) (-3.4013, 5.0398) (-3.2834, 5.0398) knots 0 0 0 1 2 2 2
  spline S96 degree 2 poles (-3.2834, 5.0398) (-3.1704, 5.0398) (-2.9491, 4.9851) (-2.8738, 4.9475) knots 0 0 0 1 2 2 2
  line L116 (-2.8738, 4.9475) -> (-2.8738, 4.7347)
  line L117 (-2.8738, 4.7347) -> (-2.8883, 4.7347)
  spline S97 degree 2 poles (-2.8883, 4.7347) (-2.9516, 4.7809) (-3.1655, 4.866) (-3.2712, 4.866) knots 0 0 0 1 2 2 2
  spline S98 degree 2 poles (-3.2712, 4.866) (-3.3332, 4.866) (-3.4572, 4.8271) (-3.4986, 4.7821) knots 0 0 0 1 2 2 2
  spline S99 degree 2 poles (-3.4986, 4.7821) (-3.5387, 4.7372) (-3.5812, 4.6302) (-3.5812, 4.5488) knots 0 0 0 1 2 2 2
  spline S100 degree 2 poles (-3.5812, 4.5488) (-3.5812, 4.4673) (-3.5338, 4.3616) (-3.4913, 4.3312) knots 0 0 0 1 2 2 2
  spline S101 degree 2 poles (-3.4913, 4.3312) (-3.4487, 4.3008) (-3.3332, 4.2777) (-3.2652, 4.2777) knots 0 0 0 1 2 2 2
  line L118 (-3.2652, 4.2777) -> (-3.1801, 4.2777)
  line L119 (-3.1801, 4.2777) -> (-3.1801, 4.1112)
  line L120 (-3.1801, 4.1112) -> (-3.2469, 4.1112)
  spline S102 degree 2 poles (-3.2469, 4.1112) (-3.3819, 4.1112) (-3.552, 3.9823) (-3.552, 3.8595) knots 0 0 0 1 2 2 2
  spline S103 degree 2 poles (-3.552, 3.8595) (-3.552, 3.8024) (-3.5083, 3.721) (-3.473, 3.6966) knots 0 0 0 1 2 2 2
  spline S104 degree 2 poles (-3.473, 3.6966) (-3.4353, 3.6711) (-3.343, 3.6505) (-3.2907, 3.6505) knots 0 0 0 1 2 2 2
  spline S105 degree 2 poles (-4.9451, 4.2582) (-4.9451, 4.6618) (-4.7105, 5.0398) (-4.4661, 5.0398) knots 0 0 0 1 2 2 2
  spline S106 degree 2 poles (-4.4661, 5.0398) (-4.2182, 5.0398) (-3.986, 4.6545) (-3.986, 4.2595) knots 0 0 0 1 2 2 2
  spline S107 degree 2 poles (-3.986, 4.2595) (-3.986, 3.8535) (-4.2206, 3.4778) (-4.4661, 3.4778) knots 0 0 0 1 2 2 2
  spline S108 degree 2 poles (-4.4661, 3.4778) (-4.7129, 3.4778) (-4.9451, 3.8668) (-4.9451, 4.2582) knots 0 0 0 1 2 2 2
  spline S109 degree 2 poles (-4.6874, 4.7153) (-4.7165, 4.6411) (-4.7409, 4.4126) (-4.7409, 4.2582) knots 0 0 0 1 2 2 2
  spline S110 degree 2 poles (-4.7409, 4.2582) (-4.7409, 4.1039) (-4.7165, 3.8766) (-4.6862, 3.8) knots 0 0 0 1 2 2 2
  spline S111 degree 2 poles (-4.6862, 3.8) (-4.6558, 3.7234) (-4.55, 3.6444) (-4.4661, 3.6444) knots 0 0 0 1 2 2 2
  spline S112 degree 2 poles (-4.4661, 3.6444) (-4.3823, 3.6444) (-4.2741, 3.7234) (-4.2425, 3.8024) knots 0 0 0 1 2 2 2
  spline S113 degree 2 poles (-4.2425, 3.8024) (-4.2121, 3.879) (-4.1902, 4.1124) (-4.1902, 4.2595) knots 0 0 0 1 2 2 2
  spline S114 degree 2 poles (-4.1902, 4.2595) (-4.1902, 4.4175) (-4.2097, 4.629) (-4.2413, 4.7116) knots 0 0 0 1 2 2 2
  spline S115 degree 2 poles (-4.2413, 4.7116) (-4.2704, 4.7894) (-4.3786, 4.8733) (-4.4661, 4.8733) knots 0 0 0 1 2 2 2
  spline S116 degree 2 poles (-4.4661, 4.8733) (-4.5488, 4.8733) (-4.657, 4.7943) (-4.6874, 4.7153) knots 0 0 0 1 2 2 2
  spline S117 degree 2 poles (0.5529, 3.9079) (0.6648, 3.9079) (0.8483, 3.841) (0.9128, 3.779) knots 0 0 0 1 2 2 2
  spline S118 degree 2 poles (0.9128, 3.779) (0.976, 3.7182) (1.0416, 3.5529) (1.0416, 3.4593) knots 0 0 0 1 2 2 2
  spline S119 degree 2 poles (1.0416, 3.4593) (1.0416, 3.3378) (0.9115, 3.1336) (0.7875, 3.0728) knots 0 0 0 1 2 2 2
  line L121 (0.7875, 3.0728) -> (0.7875, 3.0667)
  spline S120 degree 2 poles (0.7875, 3.0667) (0.8982, 3.0023) (1.0051, 2.8491) (1.0051, 2.7349) knots 0 0 0 1 2 2 2
  spline S121 degree 2 poles (1.0051, 2.7349) (1.0051, 2.5659) (0.7499, 2.3398) (0.5529, 2.3398) knots 0 0 0 1 2 2 2
  spline S122 degree 2 poles (0.5529, 2.3398) (0.3487, 2.3398) (0.102, 2.5537) (0.102, 2.7215) knots 0 0 0 1 2 2 2
  spline S123 degree 2 poles (0.102, 2.7215) (0.102, 2.8224) (0.2199, 3.0193) (0.3305, 3.0752) knots 0 0 0 1 2 2 2
  line L122 (0.3305, 3.0752) -> (0.3305, 3.0813)
  spline S124 degree 2 poles (0.3305, 3.0813) (0.1992, 3.1421) (0.0643, 3.3171) (0.0643, 3.4557) knots 0 0 0 1 2 2 2
  spline S125 degree 2 poles (0.0643, 3.4557) (0.0643, 3.6477) (0.3439, 3.9079) (0.5529, 3.9079) knots 0 0 0 1 2 2 2
  spline S126 degree 2 poles (0.2709, 3.4751) (0.2709, 3.3827) (0.3439, 3.2733) (0.4472, 3.2174) knots 0 0 0 1 2 2 2
  spline S127 degree 2 poles (0.4472, 3.2174) (0.4812, 3.198) (0.5955, 3.153) (0.6672, 3.1238) knots 0 0 0 1 2 2 2
  spline S128 degree 2 poles (0.6672, 3.1238) (0.7499, 3.1785) (0.8386, 3.3414) (0.8386, 3.4447) knots 0 0 0 1 2 2 2
  spline S129 degree 2 poles (0.8386, 3.4447) (0.8386, 3.5809) (0.6745, 3.7584) (0.5505, 3.7584) knots 0 0 0 1 2 2 2
  spline S130 degree 2 poles (0.5505, 3.7584) (0.4241, 3.7584) (0.2709, 3.6064) (0.2709, 3.4751) knots 0 0 0 1 2 2 2
  spline S131 degree 2 poles (0.2989, 2.7239) (0.2989, 2.623) (0.4338, 2.4881) (0.5542, 2.4881) knots 0 0 0 1 2 2 2
  spline S132 degree 2 poles (0.5542, 2.4881) (0.6636, 2.4881) (0.8034, 2.6084) (0.8034, 2.7118) knots 0 0 0 1 2 2 2
  spline S133 degree 2 poles (0.8034, 2.7118) (0.8034, 2.7859) (0.7316, 2.8892) (0.6599, 2.9306) knots 0 0 0 1 2 2 2
  spline S134 degree 2 poles (0.6599, 2.9306) (0.6295, 2.9476) (0.5007, 3.0071) (0.4484, 3.0242) knots 0 0 0 1 2 2 2
  spline S135 degree 2 poles (0.4484, 3.0242) (0.3609, 2.9573) (0.2989, 2.8151) (0.2989, 2.7239) knots 0 0 0 1 2 2 2
  spline S136 degree 2 poles (-1.0674, 3.3876) (-1.0674, 3.5031) (-0.9908, 3.6988) (-0.9264, 3.7644) knots 0 0 0 1 2 2 2
  spline S137 degree 2 poles (-0.9264, 3.7644) (-0.8595, 3.8337) (-0.6918, 3.9054) (-0.5909, 3.9054) knots 0 0 0 1 2 2 2
  spline S138 degree 2 poles (-0.5909, 3.9054) (-0.49, 3.9054) (-0.3235, 3.8374) (-0.2603, 3.7693) knots 0 0 0 1 2 2 2
  spline S139 degree 2 poles (-0.2603, 3.7693) (-0.1825, 3.6879) (-0.0949, 3.4144) (-0.0949, 3.215) knots 0 0 0 1 2 2 2
  spline S140 degree 2 poles (-0.0949, 3.215) (-0.0949, 3.0193) (-0.1752, 2.7045) (-0.259, 2.5878) knots 0 0 0 1 2 2 2
  spline S141 degree 2 poles (-0.259, 2.5878) (-0.3405, 2.4735) (-0.5982, 2.3459) (-0.7672, 2.3459) knots 0 0 0 1 2 2 2
  spline S142 degree 2 poles (-0.7672, 2.3459) (-0.817, 2.3459) (-0.9045, 2.3556) (-0.9373, 2.3665) knots 0 0 0 1 2 2 2
  line L123 (-0.9373, 2.3665) -> (-0.9373, 2.5598)
  line L124 (-0.9373, 2.5598) -> (-0.9288, 2.5598)
  spline S143 degree 2 poles (-0.9288, 2.5598) (-0.9009, 2.5452) (-0.7988, 2.5197) (-0.7404, 2.5197) knots 0 0 0 1 2 2 2
  spline S144 degree 2 poles (-0.7404, 2.5197) (-0.5532, 2.5197) (-0.3235, 2.7725) (-0.3016, 3.0205) knots 0 0 0 1 2 2 2
  spline S145 degree 2 poles (-0.3016, 3.0205) (-0.3733, 2.9707) (-0.524, 2.916) (-0.614, 2.916) knots 0 0 0 1 2 2 2
  spline S146 degree 2 poles (-0.614, 2.916) (-0.7015, 2.916) (-0.8328, 2.9512) (-0.9045, 3.0047) knots 0 0 0 1 2 2 2
  spline S147 degree 2 poles (-0.9045, 3.0047) (-0.9872, 3.0667) (-1.0674, 3.2588) (-1.0674, 3.3876) knots 0 0 0 1 2 2 2
  spline S148 degree 2 poles (-0.8632, 3.3961) (-0.8632, 3.3037) (-0.8146, 3.1785) (-0.7611, 3.1348) knots 0 0 0 1 2 2 2
  spline S149 degree 2 poles (-0.7611, 3.1348) (-0.721, 3.1032) (-0.6213, 3.0825) (-0.569, 3.0825) knots 0 0 0 1 2 2 2
  spline S150 degree 2 poles (-0.569, 3.0825) (-0.4985, 3.0825) (-0.366, 3.125) (-0.3016, 3.1652) knots 0 0 0 1 2 2 2
  spline S151 degree 2 poles (-0.3016, 3.1652) (-0.3004, 3.187) (-0.2979, 3.2284) (-0.2979, 3.26) knots 0 0 0 1 2 2 2
  spline S152 degree 2 poles (-0.2979, 3.26) (-0.2979, 3.4156) (-0.3587, 3.6064) (-0.4049, 3.6562) knots 0 0 0 1 2 2 2
  spline S153 degree 2 poles (-0.4049, 3.6562) (-0.4475, 3.7037) (-0.5398, 3.7413) (-0.5921, 3.7413) knots 0 0 0 1 2 2 2
  spline S154 degree 2 poles (-0.5921, 3.7413) (-0.7137, 3.7413) (-0.8632, 3.5687) (-0.8632, 3.3961) knots 0 0 0 1 2 2 2
  point P0 (0, 0)
  point P1 (5, -3)
  dimension "d92" = 7
  dimension "d93" = 4
  dimension "d94" = 11
  dimension "d95" = 14
  dimension "d97" = 2
  dimension "d98" = 3
  dimension "d99" = 2
  dimension "d100" = 2
  dimension "d101" = 2
  dimension "d102" = 3
  dimension "d103" = 2
  dimension "d104" = 100
  dimension "d105" = 6
  dimension "d106" = 1
  dimension "d107" = 5
  dimension "d108" = 1
  dimension "d109" = 1
  dimension "d110" = 2
  dimension "d111" = 0.5
  dimension "d112" = 1.5
  dimension "d113" = 0.1
  dimension "d115" = 0.1
  dimension "d116" = 0.1
  dimension "d117" = 0.1
  dimension "d118" = 0.1
  dimension "d120" = 0.1
  dimension "d121" = 0.1
  dimension "d122" = 0.1
  dimension "d123" = 0.1
  dimension "d124" = 0.1
  dimension "d125" = 0.9
  dimension "d126" = 1.4
  dimension "d129" = 0.1
  dimension "d131" = 2.1
  dimension "d133" = 1.9
  dimension "d134" = 1.4
  dimension "d135" = 60
  dimension "d136" = 60
  dimension "d139" = 0.1
  dimension "d140" = 0.1
  dimension "d141" = 0.1
  dimension "d142" = 2
  dimension "d143" = 0.1
  dimension "d144" = 0.1
  dimension "d145" = 0.1
  dimension "d146" = 2
  dimension "d147" = 0.1
  constraints: 114 end point, 13 horizontal, 11 parallel, 11 point on line, 10 perpendicular, 9 vertical, 3 midpoint, 2 collinear, 16 other
  measures "d92" distance of L0.start L0.end
  measures "d93" distance of L0.end L1.end
  measures "d94" distance between parallel lines of L4 L1
  measures "d95" distance between parallel lines of L2 L5
  measures "d97" distance from line of L6.end L1
  measures "d98" distance of L6.end L50.start
  measures "d99" distance between parallel lines of L8 L3
  measures "d100" distance of L7.start L7.end
  measures "d101" distance of L10.end L11.start
  measures "d102" distance of L6.start L51.start
  measures "d103" distance of L14.start L14.end
  measures "d104" angle of L15 L14
  measures "d105" distance of L15.start L15.end
  measures "d106" distance of L14.end L15.end
  measures "d107" distance of L15.end L16.end
  measures "d108" distance of L17.start L17.end
  measures "d109" distance of L19.start L19.end
  measures "d110" distance of L19.end L20.end
  measures "d111" distance from line of L17 L15.start
  measures "d112" distance of L19.start L17.start
  measures "d113" distance between parallel lines of L41 L13
  measures "d115" distance between parallel lines of L8 L45
  measures "d116" distance between parallel lines of L47 L7
  measures "d117" distance between parallel lines of L48 L7
  measures "d118" distance between parallel lines of L46 L9
  measures "d120" distance between parallel lines of L2 L52
  measures "d121" distance between parallel lines of L20 L56
  measures "d122" distance between parallel lines of L60 L18
  measures "d123" distance between parallel lines of L17 L61
  measures "d124" distance between parallel lines of L64 L16
  measures "d125" distance between parallel lines of L45 L43
  measures "d126" distance between parallel lines of L9 L52
  measures "d129" distance between parallel lines of L49 L6
  measures "d131" distance between parallel lines of L68 L55
  measures "d133" distance between parallel lines of L13 L55
  measures "d134" distance between parallel lines of L12 L54
  measures "d135" angle of L10 L69
  measures "d136" angle of L11 L70
  measures "d139" distance between parallel lines of L54 L71
  measures "d140" distance between parallel lines of L73 L72
  measures "d141" distance between parallel lines of L68 L72
  measures "d142" distance from line of L6.start L3
  measures "d143" distance between parallel lines of L52 L74
  measures "d144" distance between parallel lines of L67 L75
  measures "d145" distance between parallel lines of L77 L75
  measures "d146" distance between parallel lines of L75 L53
  measures "d147" distance between parallel lines of L78 L14
emboss "Emboss3" sketch "Sketch5" operation add depth 0.1 direction (0, 0, 1) contours L3 L2 L76 L52 L55 L54 L53 L78 L1 L0 | L0 L49 L2 L6 | L2 L1 L14 L53 L52 L76 | L78 L53 L14 L1 | L78 L63 L14 L53 | L63 L65 L15 L16 L66 L64 | L17 L18 L62 L60 L61 L15 | L11 L70 L41 L42 L68 L51 L72 L71 L73 L12 L13 L69 L10 | L7 L44 L48 L8 L9 L77 L74 L75 L50 L67 L46 L45 L47 L43 | L19 L20 L58 L56 L57 L59 | S0 S1 S2 L79 S3 S4 S5 S6 L80 S7 S8 | L81 L82 L83 L84 L85 L86 L87 | S19 S20 S21 S22 S23 S24 L88 S25 S26 S27 L89 L90 S28 S29 S30 L91 L92 L93 | S35 S36 S37 L95 S38 S39 S40 S41 L96 S42 S43 | L97 L98 L99 L100 L101 L102 L103 | S54 S55 S56 L104 S57 S58 S59 S60 L105 S61 S62 | S73 S74 S75 L106 L107 S76 S77 S78 S79 S80 S81 S82 L108 L109 L110 L111 L112 S83 S84 S85 | S86 S87 L113 L114 S88 S89 S90 S91 L115 S92 S93 S94 S95 S96 L116 L117 S97 S98 S99 S100 S101 L118 L119 L120 S102 S103 S104 | S105 S106 S107 S108 | S117 S118 S119 L121 S120 S121 S122 S123 L122 S124 S125 | S136 S137 S138 S139 S140 S141 S142 L123 L124 S143 S144 S145 S146 S147